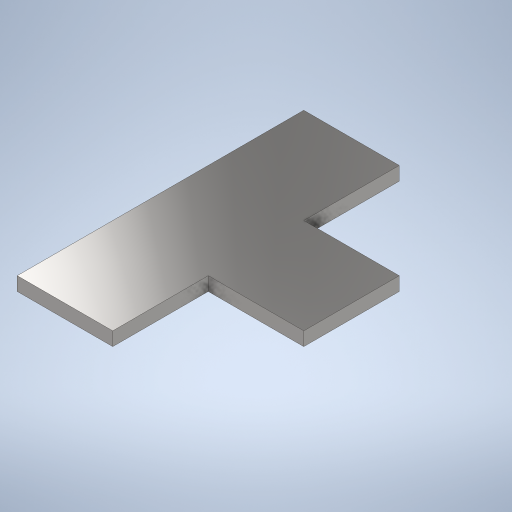
# Autodesk Inventor part: Part1
Saved by Autodesk Inventor 2023 (Build 270158000, 158)
## iProperties
Created: 2022-07-26
Part Number: Part1
Material: Steel, Mild
Document SubType Name: Sheet Metal
Designer: earls
Density: 7.85 g/cm^3
Sheet Metal Rule: Default_mm
Appearance: Semi-Polished
Author: earls
Autodesk Inventor part; units mm, degrees
ref_plane "YZ Plane" through (0, 0, 0) normal (1, 0, 0) x (0, 1, 0)
ref_plane "XZ Plane" through (0, 0, 0) normal (0, 1, 0) x (-1, 0, 0)
ref_plane "XY Plane" through (0, 0, 0) normal (0, 0, 1) x (1, 0, 0)
sketch "Sketch1" plane through (0, 0, 0) normal (0, 1, 0) x (-1, 0, 0)
  line L0 (9.3536, 7.4669) -> (2.3536, 7.4669)
  line L1 (2.3536, 7.4669) -> (2.3536, 14.4669)
  line L2 (2.3536, 14.4669) -> (-4.6464, 14.4669)
  line L3 (-4.6464, 14.4669) -> (-4.6464, 21.4669)
  line L4 (-4.6464, 21.4669) -> (2.3536, 21.4669)
  line L5 (2.3536, 21.4669) -> (2.3536, 28.4669)
  line L6 (2.3536, 28.4669) -> (9.3536, 28.4669)
  line L7 (9.3536, 28.4669) -> (9.3536, 7.4669)
  point P0 (0, 0)
  dimension "d0" = 7
  dimension "d1" = 7
  dimension "d2" = 21
  measures "d0" distance of L0.start L0.end
  measures "d1" distance of L0.end L1.end
  measures "d2" distance of L6.end L0.start
extrude "Plate1" add sketch "Sketch1" along normal blind 1
equation "\"d3\" = Thickness"
equation "\"BendRadius\" = Thickness"
equation "\"BendReliefWidth\" = Thickness"
equation "\"BendReliefDepth\" = 0.5 * Thickness"
equation "\"CornerReliefSize\" = 4 * Thickness"
equation "\"MinimumRemnant\" = 2 * Thickness"
equation "\"TransitionRadius\" = BendRadius"
equation "\"JacobiRadiusSize\" = BendRadius"
equation "\"GapSize\" = Thickness"
equation "\"Thickness\" = 1"
body "Solid1"
